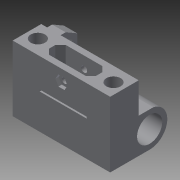
# Autodesk Inventor part: x-end-idler
Saved by Autodesk Inventor 2015 SP2 (Build 190223200, 223)
## iProperties
Created: 2015-06-01
Part Number: x-end-idler
Material: Generic
Document SubType Name: Modeling
Designer: Marc
Density: 1 g/cm^3
Appearance: Default
Author: Marc
Autodesk Inventor part; units mm, degrees
ref_plane "YZ Plane" through (0, 0, 0) normal (1, 0, 0) x (0, 1, 0)
ref_plane "XZ Plane" through (0, 0, 0) normal (0, 1, 0) x (-1, 0, 0)
ref_plane "XY Plane" through (0, 0, 0) normal (0, 0, 1) x (1, 0, 0)
sketch "Sketch1" plane through (0, 0, 0) normal (0, 1, 0) x (-1, 0, 0)
  line L0 (0, 0) -> (58, 0)
  line L1 (58, 0) -> (58, -39)
  line L2 (58, -39) -> (0, -39)
  line L3 (0, -39) -> (0, 0)
  dimension "d0" = 58
  dimension "d1" = 39
  constraints: 8 end point, 2 parallel, 1 horizontal, 1 perpendicular
  measures "d0" distance of L0.start L0.end
  measures "d1" distance of L2.end L0.start
extrude "Extrusion1" add sketch "Sketch1" along normal blind 35
sketch "Sketch2" plane through (0, 0, 0) normal (1, 0, 0) x (0, 0, -1)
  line L0 (39, 0) -> (0, 0) projected
  circle A0 centre (28.5, 23.5) radius 7.5
  arc A1 (39, 23.5) -> (18.2322, 25.6959) centre (28.5, 23.5) ccw
  line L1 (39, 0) -> (39, 35) projected
  line L2 (19.5, 23.5) -> (15.5, 16.5718)
  line L3 (15.5, 16.5718) -> (7.5, 16.5718)
  line L4 (7.5, 16.5718) -> (3.5, 23.5)
  line L5 (3.5, 23.5) -> (7.5, 30.4282)
  line L6 (7.5, 30.4282) -> (15.5, 30.4282)
  line L7 (15.5, 30.4282) -> (19.5, 23.5)
  line L8 (0, 0) -> (39, 0)
  line L9 (39, 0) -> (39, 17)
  line L10 (0, 17) -> (0, 0)
  line L11 (3.5, 23.5) -> (3.5, 17)
  line L12 (39, 23.5) -> (39, 17)
  line L13 (3.5, 17) -> (0, 17)
  line L14 (15.5, 16.5718) -> (7.5, 16.5718)
  point P0 (11.5, 23.5)
  point P1 (11.5, 23.5)
  dimension "d5" = 15
  dimension "d6" = 3
  dimension "d8" = 8
  dimension "d13" = 23.5
  dimension "d14" = 17
  dimension "d71" = 6.5
  dimension "d72" = 17
  constraints: 26 end point, 4 parallel, 3 perpendicular, 3 point on line, 2 centre point, 2 collinear, 2 point on circle, 2 tangent, 1 coincident, 1 horizontal, 13 other
  measures "d5" diameter of A0
  measures "d6" radial gap between concentric circles of A1 A0
  measures "d8" distance of L5.end L6.end
  measures "d13" distance from line of L0 A0.centre
  measures "d14" distance between parallel lines of L0 L13
  measures "d71" distance from line of L13 point (11.5, 23.5)
  measures "d72" distance of A0.centre point (11.5, 23.5)
extrude "Extrusion2" cut sketch "Sketch2" against normal through all keep common part
sketch "Sketch3" plane through (0, 17, -3.5) normal (0, 0, 1) x (1, 0, 0)
  line L0 (-50, 0) -> (0, 0)
  line L1 (0, 0) -> (0, 13.4282)
  line L2 (0, 13.4282) -> (-50, 13.4282)
  line L3 (-50, 13.4282) -> (-50, 0)
  line L4 (0, 0) -> (-58, 0) projected
  line L5 (0, 0) -> (0, 6.5) projected
  line L6 (0, 13.4282) -> (-58, 13.4282) projected
  line L7 (-58, 6.5) -> (-58, 0) projected
  point P0 (0, -17)
  dimension "d18" = 8
  constraints: 8 end point, 3 collinear, 2 parallel, 1 horizontal, 1 perpendicular
  measures "d18" distance between parallel lines of L7 L3
extrude "Extrusion3" cut sketch "Sketch3" against normal up to surface (14.7322 mm away)
sketch "Sketch4" plane through (-58, 17, 0) normal (0, 1, 0) x (1, 0, 0)
  line L0 (44, 18.2322) -> (16, 18.2322)
  line L1 (16, 18.2322) -> (16, 17.2322)
  line L2 (16, 17.2322) -> (44, 17.2322)
  line L3 (44, 17.2322) -> (44, 18.2322)
  line L4 (58, 18.2322) -> (58, 0) projected
  line L5 (58, 18.2322) -> (8, 18.2322) projected
  dimension "d21" = 1
  dimension "d22" = 28
  dimension "d23" = 14
  constraints: 8 end point, 2 parallel, 1 collinear, 1 horizontal, 1 perpendicular
  measures "d21" distance of L2.end L0.start
  measures "d22" distance of L1.end L2.end
  measures "d23" distance between parallel lines of L4 L3
extrude "Extrusion4" cut sketch "Sketch4" against normal through all
sketch "Sketch5" plane through (-58, 0, 0) normal (0, 0, 1) x (1, 0, 0)
  line L0 (18.071, 13.5) -> (15, 10.429)
  line L1 (15, 10.429) -> (15, 6.571)
  line L2 (16, 17) -> (16, 0) projected
  line L3 (15, 6.571) -> (18.071, 3.5)
  line L4 (18.071, 3.5) -> (39.929, 3.5)
  line L5 (39.929, 3.5) -> (43, 6.571)
  line L6 (43, 6.571) -> (43, 10.429)
  line L7 (43, 10.429) -> (39.929, 13.5)
  line L8 (39.929, 13.5) -> (18.071, 13.5)
  line L9 (0, 0) -> (58, 0) projected
  line L10 (29, 13.5) -> (29, 3.5) construction
  line L11 (58, 0) -> (58, 17) projected
  dimension "d26" = 10
  dimension "d27" = 28
  dimension "d28" = 3.5
  dimension "d29" = 135
  dimension "d30" = 135
  dimension "d31" = 3.858
  dimension "d32" = 29
  constraints: 18 end point, 5 perpendicular, 4 parallel, 2 midpoint
  measures "d26" distance between parallel lines of L4 L8
  measures "d27" distance between parallel lines of L6 L1
  measures "d28" distance between parallel lines of L9 L4
  measures "d29" angle of L7 L8
  measures "d30" angle of L4 L5
  measures "d31" distance of L5.end L6.end
  measures "d32" distance between parallel lines of L11 L10
extrude "Extrusion5" cut sketch "Sketch5" against normal through all
sketch "Sketch7" plane through (-58, 0, 0) normal (0, 0, 1) x (1, 0, 0)
  line L0 (58, 0) -> (0, 0) projected
  line L1 (29, 0) -> (29, 17) construction
  line L2 (0, 17) -> (58, 17) construction
  line L3 (6.5, 8.5) -> (51.5, 8.5) construction
  dimension "d35" = 45
  dimension "d36" = 8.5
  dimension "d37" = 22.5
  constraints: 4 end point, 2 midpoint, 1 horizontal
  measures "d35" distance of L3.end L3.start
  measures "d36" distance from line of L0 L3.end
  measures "d37" distance from line of L3.end L1
hole "Hole1" at (-51.5, 8.5, 0) at (-6.5, 8.5, 0) direction (0, 0, -1) diameter 8.5 depth 37
sketch "Sketch8" plane through (-58, 17, 0) normal (0, 1, 0) x (1, 0, 0)
  line L0 (43, 0) -> (43, 17.2322) projected
  line L1 (0, 0) -> (58, 0) projected
  point P0 (29, 7)
  dimension "d45" = 14
  dimension "d46" = 7
  measures "d45" distance from line of L0 point (29, 7)
  measures "d46" distance from line of L1 point (29, 7)
hole "Hole2" at (-29, 17, -7) direction (0, -1, 0) diameter 3.6 end through all counterbore diameter 6.2 counterbore depth 2
hole "Hole3" at (0, 23.5, -11.5) direction (-1, 0, 0) diameter 5.7 end through all
sketch "Sketch9" plane through (0, 0, 0) normal (0, -1, 0) x (1, 0, 0)
  line L0 (-27.2, -3.8823) -> (-25.4, -7)
  line L1 (-25.4, -7) -> (-27.2, -10.1177)
  line L2 (-27.2, -10.1177) -> (-30.8, -10.1177)
  line L3 (-30.8, -10.1177) -> (-32.6, -7)
  line L4 (-32.6, -7) -> (-30.8, -3.8823)
  line L5 (-30.8, -3.8823) -> (-27.2, -3.8823)
  circle A0 centre (-29, -7) radius 1.8 projected
  point P0 (0, 0)
  dimension "d63" = 3.6
  constraints: 12 end point, 1 coincident, 1 horizontal, 13 other
  measures "d63" distance of L1.end L2.end
extrude "Extrusion6" cut sketch "Sketch9" against normal blind 2
sketch "Sketch10" plane through (-50, 17, -3.5) normal (1, 0, 0) x (0, 0, -1)
  line L0 (10.25, 10.3971) -> (12.5, 6.5)
  line L1 (12.5, 6.5) -> (10.25, 2.6029)
  line L2 (10.25, 2.6029) -> (5.75, 2.6029)
  line L3 (5.75, 2.6029) -> (3.5, 6.5)
  line L4 (3.5, 6.5) -> (5.75, 10.3971)
  line L5 (5.75, 10.3971) -> (10.25, 10.3971)
  circle A0 centre (8, 6.5) radius 2.85
  circle A1 centre (8, 6.5) radius 2.85 projected
  line L6 (4, 13.4282) -> (12, 13.4282) projected
  point P0 (-3.5, -17)
  dimension "d66" = 4.5
  constraints: 12 end point, 2 concentric, 1 centre point, 1 coincident, 1 parallel, 13 other
  measures "d66" distance of L4.end L0.start
extrude "Extrusion7" cut sketch "Sketch10" against normal blind 5
equation "\"d59\" = d13"
body "Solid1"
